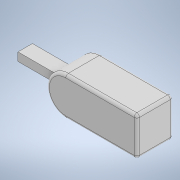
# Autodesk Inventor part: bat_sketch
Saved by Autodesk Inventor 2020 (Build 240168000, 168)
## iProperties
Created: 2023-12-20
Part Number: bat_sketch
Material: Типовые
Document SubType Name: Modeling
Designer: denis
Density: 1 g/cm^3
Appearance: По умолчанию
Author: denis
Autodesk Inventor part; units mm, degrees
ref_plane "YZ Plane" through (0, 0, 0) normal (1, 0, 0) x (0, 1, 0)
ref_plane "XZ Plane" through (0, 0, 0) normal (0, 1, 0) x (-1, 0, 0)
ref_plane "XY Plane" through (0, 0, 0) normal (0, 0, 1) x (1, 0, 0)
sketch "Эскиз1" plane through (0, 0, 0) normal (0, 0, 1) x (1, 0, 0)
  line L0 (0, 0) -> (-52, 0)
  line L1 (-52, 0) -> (-52, -28) construction
  line L2 (-52, -28) -> (0, -28)
  line L3 (0, -28) -> (0, 0)
  arc A0 (-52, 0) -> (-52, -28) centre (-52, -14) ccw
  point P0 (-66, -14)
  dimension "d1" = 28
  dimension "d2" = 66
  constraints: 8 end point, 3 point on circle, 2 parallel, 1 centre point, 1 horizontal, 1 midpoint, 1 perpendicular
  measures "d1" distance of L2.end L0.start
  measures "d2" distance from line of L3 point (-66, -14)
extrude "Выдавливание1" add sketch "Эскиз1" along normal blind 26.5
fillet "Сопряжение1" radius 2 2 edges at (0, -14, 26.5) (0, -14, 0)
fillet "Сопряжение2" radius 2 12 edges at (-0.5858, 0, 25.9142) (-27, 0, 26.5) (-66, -14, 26.5) (-27, -28, 26.5) (-0.5858, -28, 25.9142) (0, -28, 13.25) (-0.5858, -28, 0.5858) (-27, -28, 0) (-66, -14, 0) (-27, 0, 0) (-0.5858, 0, 0.5858) (0, 0, 13.25)
sketch "Эскиз2" plane through (0, -26, 24.5) normal (1, 0, 0) x (0, 0, -1)
  line L0 (6.0366, 15.0348) -> (16.61, 15.0348)
  line L1 (16.61, 15.0348) -> (16.61, 8.9331)
  line L2 (16.61, 8.9331) -> (6.0366, 8.9331)
  line L3 (6.0366, 8.9331) -> (6.0366, 15.0348)
  point P0 (24.5, 26)
  constraints: 8 end point, 2 parallel, 1 horizontal, 1 perpendicular
extrude "Выдавливание2" add sketch "Эскиз2" against normal blind 95
